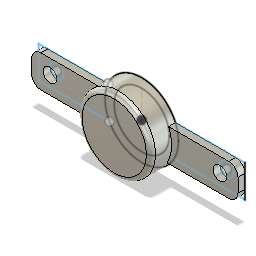
Intake+Bearing+Cap (Autodesk Fusion 360 design; units mm, degrees)
Autodesk Fusion 360 part; units mm, degrees
sketch "Sketch1" plane through (0, 0, 0) normal (0, 0, 1) x (1, 0, 0)
  circle A0 centre (0, 0) radius 15.24
  circle A1 centre (0, 0) radius 20.32
  line L0 (18.6388, 8.093) -> (57.15, 8.093)
  line L1 (57.15, 8.093) -> (57.15, -9.687)
  line L2 (57.15, -9.687) -> (17.8624, -9.687)
  line L3 (0, 15.24) -> (0, -15.24) construction
  line L4 (-18.6388, 8.093) -> (-57.15, 8.093)
  line L5 (-57.15, 8.093) -> (-57.15, -9.687)
  line L6 (-57.15, -9.687) -> (-17.8624, -9.687)
  circle A2 centre (-47.1067, 0) radius 3.81
  circle A3 centre (47.1067, 0) radius 3.81
  dimension "d1" = 30.48
  dimension "d2" = 5.08
  dimension "d3" = 57.15
  dimension "d4" = 17.78
  dimension "d11" = 7.62
  constraint coincident A0.centre A1.centre
  constraint horizontal L0
  constraint vertical L1
  constraint horizontal L2
  constraint coincident A1 L0.start
  constraint coincident A1 L2.end
  constraint coincident A0 L3.start
  constraint coincident A0 L3.end
  constraint perpendicular L0 L3
  constraint symmetric L0.start L3 L4.start
  constraint symmetric L0.end L3 L4.end
  constraint symmetric L1.end L3 L5.end
  constraint symmetric L2.end L3 L6.end
  constraint symmetric L3 A2 A3
  measures "d1" diameter of A0
  measures "d3" distance of A0.centre L1
  measures "d4" distance of L0 L2
  measures "d11" diameter of A2
extrude "Extrude1" add sketch "Sketch1" along normal blind 15.24 contours A0 | A1
extrude "Extrude2" add sketch "Sketch1" along normal blind 3.81 contours A1 L0 L1 L2 | A1 L4 L5 L6 | A2 | A3
fillet "Fillet1" radius 5.08 4 edges at (57.15, 8.093, 1.905) (57.15, -9.687, 1.905) (-57.15, 8.093, 1.905) (-57.15, -9.687, 1.905)
extrude "Extrude3" cut sketch "Sketch1" along normal blind 5.08 contours A2 | A3
extrude "Extrude4" cut sketch "Sketch1" along normal blind 10.16 contours A0
fillet "Fillet2" radius 2.54 1 edges at (-18.9449, -7.348, 15.24)
